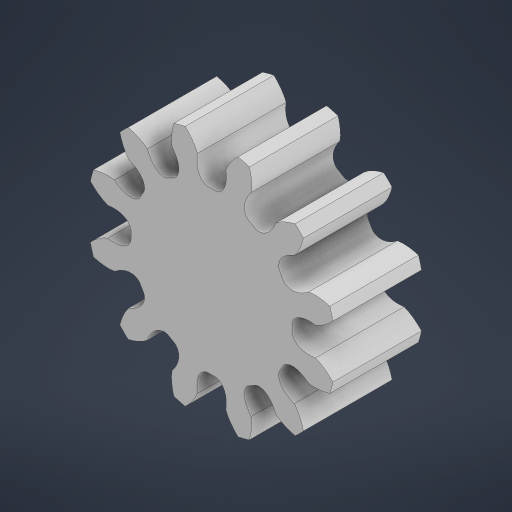
# Autodesk Inventor part: Bio12t
Saved by Autodesk Inventor 2024.1 (Build 281209000, 209)
## iProperties
Created: 2023-11-14
Part Number: Bio12t
Material: Generic
Document SubType Name: Modeling
Designer: Brandon
Density: 1 g/cm^3
Appearance: Default
Author: Brandon
Autodesk Inventor part; units mm, degrees
ref_plane "YZ Plane" through (0, 0, 0) normal (1, 0, 0) x (0, 1, 0)
ref_plane "XZ Plane" through (0, 0, 0) normal (0, 1, 0) x (-1, 0, 0)
ref_plane "XY Plane" through (0, 0, 0) normal (0, 0, 1) x (1, 0, 0)
sketch "Sketch1" plane through (0, 0, 0) normal (0, 0, 1) x (1, 0, 0)
  spline S0 degree 3 poles (-1.1349, 5.2119) (-1.1074, 5.185) (-1.0524, 5.1313) (-0.9744, 5.0464) (-0.8999, 4.9583) (-0.8297, 4.8668) (-0.7645, 4.7717) (-0.7049, 4.6729) (-0.6613, 4.5872) (-0.6305, 4.5167) (-0.6177, 4.4805) (-0.6113, 4.4624) knots 0 0 0 0 0.011529 0.023058 0.034587 0.046116 0.057645 0.069173 0.0807 0.086465 0.092229 0.092229 0.092229 0.092229
  spline S1 degree 3 poles (-0.6113, 4.4624) (-0.6155, 4.4339) (-0.624, 4.3769) (-0.6308, 4.2907) (-0.6327, 4.2043) (-0.6308, 4.1179) (-0.622, 4.0319) (-0.6073, 3.9467) (-0.5851, 3.8631) (-0.5552, 3.7819) (-0.5159, 3.7048) (-0.4749, 3.6453) (-0.4366, 3.6023) (-0.4054, 3.5723) (-0.3718, 3.5452) (-0.3356, 3.5214) (-0.2974, 3.5013) (-0.2572, 3.4852) (-0.2154, 3.4739) (-0.1727, 3.4669) (-0.1295, 3.4646) (-0.072, 3.4669) (0, 3.4676) (0.072, 3.4669) (0.1295, 3.4646) (0.1727, 3.4669) (0.2154, 3.4739) (0.2572, 3.4852) (0.2974, 3.5013) (0.3356, 3.5214) (0.3718, 3.5452) (0.4054, 3.5723) (0.4366, 3.6023) (0.4749, 3.6453) (0.5159, 3.7048) (0.5552, 3.7819) (0.5851, 3.8631) (0.6073, 3.9467) (0.622, 4.0319) (0.6308, 4.1179) (0.6327, 4.2043) (0.6308, 4.2907) (0.624, 4.3769) (0.6155, 4.4339) (0.6113, 4.4624) knots 0 0 0 0 0.008637 0.017275 0.025913 0.03455 0.043187 0.051825 0.060461 0.069097 0.077733 0.086367 0.090686 0.095003 0.099321 0.103639 0.107958 0.112278 0.116596 0.120912 0.125228 0.129548 0.138185 0.146822 0.151142 0.155458 0.159774 0.164093 0.168413 0.172731 0.177049 0.181367 0.185684 0.190003 0.198637 0.207273 0.215909 0.224545 0.233183 0.24182 0.250457 0.259095 0.267733 0.27637 0.27637 0.27637 0.27637
  spline S2 degree 3 poles (0.6113, 4.4624) (0.6177, 4.4805) (0.6305, 4.5167) (0.6613, 4.5872) (0.7049, 4.6729) (0.7645, 4.7717) (0.8297, 4.8668) (0.8999, 4.9583) (0.9744, 5.0464) (1.0524, 5.1313) (1.1074, 5.185) (1.1349, 5.2119) knots 0 0 0 0 0.005764 0.011529 0.023056 0.034584 0.046112 0.057641 0.06917 0.0807 0.092229 0.092229 0.092229 0.092229
  circle A0 centre (0, 0) radius 3.4673 construction
  circle A1 centre (0, 0) radius 4.4264 construction
  circle A2 centre (0, 0) radius 4.572 construction
  circle A3 centre (0, 0) radius 5.334
  point P0 (-1.0532, 5.1306)
  point P1 (-0.975, 5.0458)
  point P2 (-0.9006, 4.9577)
  point P3 (-0.8305, 4.8662)
  point P4 (-0.7654, 4.771)
  point P5 (-0.7061, 4.6722)
  point P6 (-0.6539, 4.5694)
  point P7 (-0.6311, 4.5165)
  point P8 (-0.623, 4.3768)
  point P9 (-0.63, 4.2907)
  point P10 (-0.632, 4.2043)
  point P11 (-0.6297, 4.118)
  point P12 (-0.621, 4.0321)
  point P13 (-0.6061, 3.947)
  point P14 (-0.5838, 3.8635)
  point P15 (-0.5537, 3.7826)
  point P16 (-0.5143, 3.7058)
  point P17 (-0.4649, 3.6349)
  point P18 (-0.4362, 3.6027)
  point P19 (-0.405, 3.5728)
  point P20 (-0.3714, 3.5457)
  point P21 (-0.3353, 3.522)
  point P22 (-0.297, 3.502)
  point P23 (-0.2569, 3.486)
  point P24 (-0.2152, 3.4746)
  point P25 (-0.1726, 3.4677)
  point P26 (-0.1296, 3.4653)
  point P27 (-0.0864, 3.4662)
  point P28 (0, 3.4673)
  point P29 (0.0864, 3.4662)
  point P30 (0.1296, 3.4653)
  point P31 (0.1726, 3.4677)
  point P32 (0.2152, 3.4746)
  point P33 (0.2569, 3.486)
  point P34 (0.297, 3.502)
  point P35 (0.3353, 3.522)
  point P36 (0.3714, 3.5457)
  point P37 (0.405, 3.5728)
  point P38 (0.4362, 3.6027)
  point P39 (0.4649, 3.6349)
  point P40 (0.5143, 3.7058)
  point P41 (0.5537, 3.7826)
  point P42 (0.5838, 3.8635)
  point P43 (0.6061, 3.947)
  point P44 (0.621, 4.0321)
  point P45 (0.6297, 4.118)
  point P46 (0.632, 4.2043)
  point P47 (0.63, 4.2907)
  point P48 (0.623, 4.3768)
  point P49 (0.6311, 4.5165)
  point P50 (0.6539, 4.5694)
  point P51 (0.7061, 4.6722)
  point P52 (0.7654, 4.771)
  point P53 (0.8305, 4.8662)
  point P54 (0.9006, 4.9577)
  point P55 (0.975, 5.0458)
  point P56 (1.0532, 5.1306)
  constraints: 4 centre point, 2 point on circle, 129 other
extrude "Extrusion1" add sketch "Sketch1" against normal blind 3.81
extrude "Extrusion2" cut sketch "Sketch1" against normal through all contours A3 S2 S1 S0 picked at (0.127, 4.7484)
pattern_circular "Circular Pattern1" count 12 over 360 about axis through (0, 0, 0) along (0, 0, -1) of "Extrusion2"
equation "\"d0\" = FaceWidth"
equation "\"Module\" = 0.762"
equation "\"PressureAngle\" = 14.5deg"
equation "\"UnitProfileClearance\" = 0.25"
equation "\"UnitRoundRadius\" = 0.3335"
equation "\"HeadDiameter\" = 10.668"
equation "\"RootDiameter\" = 6.93466"
equation "\"BaseDiameter\" = 8.85274"
equation "\"PitchDiameter\" = 9.144"
equation "\"FaceWidth\" = 3.81"
equation "\"HelixAngle\" = 0"
equation "\"UnitCorrection\" = 0"
equation "\"UnitAddendumModification\" = 0"
equation "\"CircularPitch\" = 2.39389"
equation "\"UnitBacklashShift\" = -0.199696"
equation "\"TotalToolShift\" = -0.15217"
equation "\"IsInternal\" = 0"
body "Solid1"
